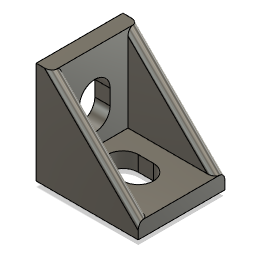
Cantoneira 20x20x17 (Autodesk Fusion 360 design; units mm, degrees)
Autodesk Fusion 360 part; units mm, degrees
sketch "Sketch1" plane through (0, 0, 0) normal (0, 0, 1) x (1, 0, 0)
  line L0 (10, -10) -> (-10, -10)
  line L1 (-10, -10) -> (-10, 10)
  line L2 (-10, 10) -> (10, 10)
  line L3 (10, 10) -> (10, -10)
  line L4 (10, -10) -> (-10, 10) construction
  line L5 (-10, -10) -> (10, 10) construction
  line L6 (-7, 10) -> (10, 10)
  line L7 (10, 10) -> (10, -7)
  line L8 (10, -7) -> (-7, -7)
  line L9 (-7, -7) -> (-7, 10)
  dimension "d1" = 20
  dimension "d2" = 20
  dimension "d3" = 3
  dimension "d4" = 3
  constraint horizontal L0
  constraint perpendicular L0 L1
  constraint parallel L0 L2
  constraint parallel L1 L3
  constraint coincident L4 origin
  constraint coincident L5 origin
  constraint horizontal L6
  constraint vertical L7
  constraint horizontal L8
  constraint vertical L9
  constraint coincident L3 L7.end
  constraint coincident L2 L6.start
  measures "d1" distance of L1.end L2.end
  measures "d2" distance of L0.end L1.end
  measures "d3" distance of L1 L9
  measures "d4" distance of L0 L8
extrude "Extrude1" add sketch "Sketch1" along normal blind 17 contours L0 L1 L2 L3 L8 L9
sketch "Sketch2" plane through (0, 0, 17) normal (0, 0, 1) x (1, 0, 0)
  line L0 (10, -7) -> (-7, -7)
  line L1 (-7, -7) -> (-7, 10)
  line L2 (-7, 10) -> (-10, 10)
  line L3 (-10, 10) -> (-10, -10)
  line L4 (-10, -10) -> (10, -10)
  line L5 (10, -10) -> (10, -7)
  line L6 (-7, 10) -> (10, -7)
  constraint coincident L1.end L2.start
  constraint coincident L0.start L5.end
extrude "Extrude2" add sketch "Sketch2" against normal blind 2 contours L0 L1 L6
sketch "Sketch3" plane through (0, 0, 0) normal (0, 0, -1) x (-1, 0, 0)
  line L0 (7, -7) -> (-10, -7)
  line L1 (-10, -7) -> (-10, -10)
  line L2 (-10, -10) -> (10, -10)
  line L3 (10, -10) -> (10, 10)
  line L4 (10, 10) -> (7, 10)
  line L5 (7, 10) -> (7, -7)
  line L6 (7, 10) -> (-10, -7)
  constraint coincident L4.end L5.start
  constraint coincident L0.end L1.start
extrude "Extrude3" add sketch "Sketch3" against normal blind 2 contours L0 L5 L6
sketch "Sketch4" plane through (-10, 0, 0) normal (-1, 0, 0) x (0, 0, 1)
  line L0 (0, 10) -> (0, -10)
  line L1 (0, -10) -> (17, -10)
  line L2 (17, -10) -> (17, 10)
  line L3 (17, 10) -> (0, 10)
  line L4 (8.5, 10) -> (8.5, -10) construction
  line L5 (11.5, -1.5) -> (11.5, 1.5)
  arc A0 (11.5, 1.5) -> (5.5, 1.5) centre (8.5, 1.5) ccw
  line L6 (5.5, 1.5) -> (5.5, -1.5)
  arc A1 (5.5, -1.5) -> (11.5, -1.5) centre (8.5, -1.5) ccw
  line L7 (8.5, -1.5) -> (8.5, 1.5) construction
  point P0 (8.5, 0)
  dimension "d11" = 6
  dimension "d12" = 3
  constraint midpoint L3 L4.start
  constraint midpoint L1 L4.end
  constraint tangent L5 A0
  constraint tangent A0 L6
  constraint parallel L5 L6
  constraint tangent L6 A1
  constraint tangent L5 A1
  constraint parallel L4 L7
  constraint coincident L4 A1.centre
  constraint midpoint L7 P0
  constraint midpoint L4 P0
  measures "d11" diameter of A0
  measures "d12" distance of A1.centre A0.centre
extrude "Extrude4" cut sketch "Sketch4" against normal through all contours L5 A0 L6 A1
ref_plane "WorkPlane1" through (-2.9289, -2.9289, 8.5) normal (-0.707107, 0.707107, 0) x (-0.707107, -0.707107, 0)
mirror "Mirror1" about plane through (-2.9289, -2.9289, 8.5) normal (-0.707107, 0.707107, 0) of "Extrude4"
sketch "Sketch5" plane through (10, 0, 0) normal (1, 0, 0) x (0, 0, -1)
  line L0 (0, -10) -> (0, -7)
  line L1 (0, -7) -> (-2, -7)
  line L2 (-2, -7) -> (-15, -7)
  line L3 (-15, -7) -> (-17, -7)
  line L4 (-17, -7) -> (-17, -10)
  line L5 (-17, -10) -> (0, -10)
  line L6 (-10.5, -10) -> (-6.5, -10)
  line L7 (-6.5, -10) -> (-6.5, -11)
  line L8 (-6.5, -11) -> (-10.5, -11)
  line L9 (-10.5, -11) -> (-10.5, -10)
  line L10 (-8.5, -10) -> (-8.5, -13.1566) construction
  point P0 (18.7716, -9.9206)
  point P1 (20.3206, -9.9206)
  point P2 (20.3206, -10.885)
  point P3 (21.7819, -10.885)
  point P4 (21.7819, -9.9206)
  dimension "d16" = 4
  dimension "d17" = 1
  dimension "d18" = 2
  constraint horizontal L6
  constraint vertical L7
  constraint horizontal L8
  constraint vertical L9
  constraint coincident L5 L6.start
  constraint midpoint L5 L10.start
  constraint perpendicular L5 L10
  measures "d16" distance of L6.start L6.end
  measures "d17" distance of L6.start L8.end
  measures "d18" distance of L7 L10
extrude "Extrude5" add sketch "Sketch5" against normal blind 20 contours L5 L6 L7 L8 L9
mirror "Mirror2" about plane through (-2.9289, -2.9289, 8.5) normal (-0.707107, 0.707107, 0) of "Extrude5"
sketch "Sketch6" plane through (0, 0, 17) normal (0, 0, 1) x (1, 0, 0)
  line L0 (10, -7) -> (-7, 10)
  line L1 (-7, 10) -> (-10, 10)
  line L2 (-10, 10) -> (-10, -10)
  line L3 (-10, -10) -> (10, -10)
  line L4 (10, -10) -> (10, -7)
  line L5 (-10, -10) -> (-8.5, -10)
  line L6 (-8.5, -10) -> (-8.5, -11.7689)
  line L7 (-8.5, -11.7689) -> (-10, -11.7689)
  line L8 (-10, -11.7689) -> (-10, -10)
  line L9 (10, -10) -> (8.5, -10)
  line L10 (8.5, -10) -> (8.5, -12.6908)
  line L11 (8.5, -12.6908) -> (10, -12.6908)
  line L12 (10, -12.6908) -> (10, -10)
  line L13 (-8.5, -10) -> (-7, -10)
  line L14 (-7, -10) -> (-7, -12.5621)
  line L15 (-7, -12.5621) -> (-8.5, -12.5621)
  line L16 (-8.5, -12.5621) -> (-8.5, -10)
  line L17 (8.5, -10) -> (7, -10)
  line L18 (7, -10) -> (7, -11.8911)
  line L19 (7, -11.8911) -> (8.5, -11.8911)
  line L20 (8.5, -11.8911) -> (8.5, -10)
  line L21 (-7, -12.5621) -> (7, -11.8911)
  dimension "d23" = 1.5
  dimension "d24" = 1.5
  dimension "d25" = 1.5
  dimension "d26" = 1.5
  constraint horizontal L5
  constraint vertical L6
  constraint horizontal L7
  constraint vertical L8
  constraint coincident L2.end L3.start
  constraint horizontal L9
  constraint vertical L10
  constraint horizontal L11
  constraint vertical L12
  constraint coincident L3.end L4.start
  constraint horizontal L13
  constraint vertical L14
  constraint horizontal L15
  constraint vertical L16
  constraint horizontal L17
  constraint vertical L18
  constraint horizontal L19
  constraint vertical L20
  measures "d23" distance of L2.end L5.end
  measures "d24" distance of L3.end L9.end
  measures "d25" distance of L5.end L13.end
  measures "d26" distance of L9.end L17.end
extrude "Extrude6" cut sketch "Sketch6" against normal through all contours L3 L9 L10 L11 L12 L20 | L3 L5 L6 L7 L8 L16 | L3 L14 L18 L21
mirror "Mirror3" about plane through (-2.9289, -2.9289, 8.5) normal (-0.707107, 0.707107, 0) of "Extrude6"
fillet "Fillet1" radius 1 4 edges at (1.5, 1.5, 17) (1.5, 1.5, 15) (1.5, 1.5, 2) (1.5, 1.5, 0)
equation "d4 = d3"
equation "d18 = d16 / 2"
